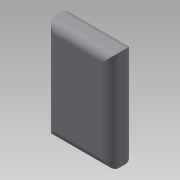
# Autodesk Inventor part: Anker
Saved by Autodesk Inventor 2015 (Build 190159000, 159)
## iProperties
Created: 2015-10-14
Part Number: Anker
Material: Generisch
Document SubType Name: Modeling
Designer: Bene
Density: 1 g/cm^3
Appearance: Vorgabe
Author: Bene
Autodesk Inventor part; units mm, degrees
ref_plane "YZ Plane" through (0, 0, 0) normal (1, 0, 0) x (0, 1, 0)
ref_plane "XZ Plane" through (0, 0, 0) normal (0, 1, 0) x (-1, 0, 0)
ref_plane "XY Plane" through (0, 0, 0) normal (0, 0, 1) x (1, 0, 0)
sketch "Skizze1" plane through (0, 0, 0) normal (0, 0, 1) x (1, 0, 0)
  line L0 (0, 0) -> (-62, 0)
  line L1 (-62, 0) -> (-62, 23)
  line L2 (-62, 23) -> (0, 23)
  line L3 (0, 23) -> (0, 0)
  dimension "d0" = 62
  dimension "d1" = 23
  constraints: 8 end point, 2 parallel, 1 horizontal, 1 perpendicular
  measures "d0" distance of L1.end L2.end
  measures "d1" distance of L0.end L1.end
extrude "Extrusion1" add sketch "Skizze1" along normal blind 96.5
sketch "Skizze2" plane through (-62, 23, 0) normal (0, 1, 0) x (1, 0, 0)
  circle A0 centre (31, -78.5) radius 7.0477
  line L0 (62, -96.5) -> (0, -96.5) projected
  line L1 (0, 0) -> (0, -96.5) projected
  point P0 (62, 0)
  dimension "d4" = 18
  dimension "d5" = 31
  constraints: 1 centre point
  measures "d4" distance from line of L0 A0.centre
  measures "d5" distance from line of A0.centre L1
extrude "Extrusion2" cut sketch "Skizze2" against normal blind 10
fillet "Rundung1" radius 8 8 edges at (0, 23, 48.25) (0, 0, 48.25) (-62, 23, 48.25) (-62, 0, 48.25) (-31, 0, 96.5) (-31, 23, 96.5) (-31, 23, 0) (-31, 0, 0)
sketch "Skizze3" plane through (0, 0, 96.5) normal (0, 0, 1) x (1, 0, 0)
  line L0 (0, 8) -> (-62, 8) projected
  line L1 (0, 8) -> (0, 15) projected
  line L2 (-62, 15) -> (0, 15) projected
  line L3 (-62, 15) -> (-62, 8) projected
  line L4 (-57.1154, 17.1012) -> (-5.8036, 17.1012)
  line L5 (-5.8036, 17.1012) -> (-5.8036, 6.3302)
  line L6 (-5.8036, 6.3302) -> (-57.1154, 6.3302)
  line L7 (-57.1154, 6.3302) -> (-57.1154, 17.1012)
  point P0 (0, 0)
  constraints: 8 end point, 2 parallel, 1 horizontal, 1 perpendicular
extrude "Extrusion3" cut sketch "Skizze3" against normal blind 10 contours L5 L6 L7 L0 | L0 L7 L2 L5 | L2 L7 L4 L5
